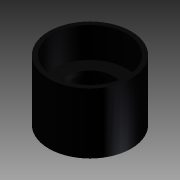
# Autodesk Inventor part: MU_Bearing_Retainer
Saved by Autodesk Inventor 2011 SP2 (Build 150309200, 309)
## iProperties
Created: 2012-02-14
Part Number: MU_Bearing_Retainer
Document SubType Name: Modeling
Designer: sungwook
Density: 2.71 g/cm^3
Material: Aluminum-6061
Mass: 0.0265628 g
Surface Area: 0.761522 cm^2
Volume: 0.00980177 cm^3
Author: sungwook
Autodesk Inventor part; units mm, degrees
ref_plane "YZ Plane" through (0, 0, 0) normal (1, 0, 0) x (0, 1, 0)
ref_plane "XZ Plane" through (0, 0, 0) normal (0, 1, 0) x (-1, 0, 0)
ref_plane "XY Plane" through (0, 0, 0) normal (0, 0, 1) x (1, 0, 0)
sketch "Sketch1" plane through (0, 0, 0) normal (0, 0, 1) x (1, 0, 0)
  circle A0 centre (0, 0) radius 1.9
  dimension "d0" = 3.8
  constraints: 1 centre point, 1 coincident
  measures "d0" diameter of A0
extrude "Extrusion1" add sketch "Sketch1" along normal blind 1.8
hole "Hole1" at (0, 0, 1.8) direction (0, 0, -1) diameter 3.4 depth 1.4
sketch "Sketch2" plane through (0, 0, 0) normal (0, 0, -1) x (-1, 0, 0)
  circle A0 centre (0, 0) radius 1.9 projected
  circle A1 centre (0, 0) radius 1.9
  dimension "d12" = 3.8
  constraints: 1 centre point, 1 coincident
  measures "d12" diameter of A1
extrude "Extrusion2" add sketch "Sketch2" along normal blind 1
hole "Hole2" at (0, 0, -1) direction (0, 0, 1) diameter 2.2 end through all
hole "Hole3" at (0, 0, -1) direction (0, 0, 1) diameter 3 depth 1.2
body "Solid1"
